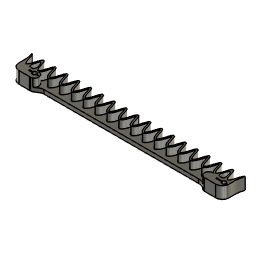
I2process_waku_8mm_change (Autodesk Fusion 360 design; units mm, degrees)
Autodesk Fusion 360 part; units mm, degrees
(part 1 of 7)
sketch "スケッチ1" plane through (0, 0, 0) normal (0, 0, 1) x (1, 0, 0)
  line L0 (269.5, 8.5) -> (265, 8.5)
  line L1 (265, 8.5) -> (262.5, 6)
  line L2 (262.5, 6) -> (257.5, 6)
  line L3 (257.5, 6) -> (255, 8.5)
  line L4 (255, 8.5) -> (250.5, 8.5)
  line L5 (250.5, 7.5) -> (255, 7.5)
  line L6 (255, 7.5) -> (257.5, 5)
  line L7 (257.5, 5) -> (262.5, 5)
  line L8 (262.5, 5) -> (265, 7.5)
  line L9 (265, 7.5) -> (269.5, 7.5)
  line L10 (269.5187, 10.492) -> (262.5532, 10.492)
  line L11 (257.4467, 10.492) -> (250.4813, 10.492)
  line L12 (250.4813, 9.5109) -> (257.4466, 9.5109)
  line L13 (262.5533, 9.5109) -> (269.5187, 9.5109)
  arc A0 (257.4466, 9.5109) -> (262.5533, 9.5109) centre (260, 10.0015) ccw
  arc A1 (262.5532, 10.492) -> (257.4467, 10.492) centre (260, 10.0015) ccw
  spline S0 degree 5 poles (10, 15) (10.1382, 15.0986) (10.4088, 15.309) (10.7966, 15.6643) (11.2779, 16.2176) (11.8206, 17.0415) (12.3075, 17.9961) (12.7453, 19.0761) (13.1463, 20.2726) (13.5274, 21.5702) (13.9072, 22.9453) (14.3043, 24.3634) (14.7345, 25.777) (15.2088, 27.1236) (15.7302, 28.3211) (16.2937, 29.2738) (16.8886, 29.8918) (17.5, 30.1073) (18.1114, 29.8918) (18.7063, 29.2738) (19.2698, 28.3211) (19.7912, 27.1236) (20.2655, 25.777) (20.6957, 24.3634) (21.0928, 22.9453) (21.4726, 21.5702) (21.8537, 20.2726) (22.2547, 19.0761) (22.6925, 17.9961) (23.1794, 17.0415) (23.7221, 16.2176) (24.2034, 15.6643) (24.5912, 15.309) (24.8618, 15.0986) (25, 15) knots 0 0 0 0 0 0 0.033333 0.066667 0.1 0.133333 0.166667 0.2 0.233333 0.266667 0.3 0.333333 0.366667 0.4 0.433333 0.466667 0.5 0.533333 0.566667 0.6 0.633333 0.666667 0.7 0.733333 0.766667 0.8 0.833333 0.866667 0.9 0.933333 0.966667 1 1 1 1 1 1
  spline S1 degree 5 poles (25, 15) (25.1382, 15.0986) (25.4088, 15.309) (25.7966, 15.6643) (26.2779, 16.2176) (26.8206, 17.0415) (27.3075, 17.9961) (27.7453, 19.0761) (28.1463, 20.2726) (28.5274, 21.5702) (28.9072, 22.9453) (29.3043, 24.3634) (29.7345, 25.777) (30.2088, 27.1236) (30.7302, 28.3211) (31.2937, 29.2738) (31.8886, 29.8918) (32.5, 30.1073) (33.1114, 29.8918) (33.7063, 29.2738) (34.2698, 28.3211) (34.7912, 27.1236) (35.2655, 25.777) (35.6957, 24.3634) (36.0928, 22.9453) (36.4726, 21.5702) (36.8537, 20.2726) (37.2547, 19.0761) (37.6925, 17.9961) (38.1794, 17.0415) (38.7221, 16.2176) (39.2034, 15.6643) (39.5912, 15.309) (39.8618, 15.0986) (40, 15) knots 0 0 0 0 0 0 0.033333 0.066667 0.1 0.133333 0.166667 0.2 0.233333 0.266667 0.3 0.333333 0.366667 0.4 0.433333 0.466667 0.5 0.533333 0.566667 0.6 0.633333 0.666667 0.7 0.733333 0.766667 0.8 0.833333 0.866667 0.9 0.933333 0.966667 1 1 1 1 1 1
  spline S2 degree 5 poles (40, 15) (40.1382, 15.0986) (40.4088, 15.309) (40.7966, 15.6643) (41.2779, 16.2176) (41.8206, 17.0415) (42.3075, 17.9961) (42.7453, 19.0761) (43.1463, 20.2726) (43.5274, 21.5702) (43.9072, 22.9453) (44.3043, 24.3634) (44.7345, 25.777) (45.2088, 27.1236) (45.7302, 28.3211) (46.2937, 29.2738) (46.8886, 29.8918) (47.5, 30.1073) (48.1114, 29.8918) (48.7063, 29.2738) (49.2698, 28.3211) (49.7912, 27.1236) (50.2655, 25.777) (50.6957, 24.3634) (51.0928, 22.9453) (51.4726, 21.5702) (51.8537, 20.2726) (52.2547, 19.0761) (52.6925, 17.9961) (53.1794, 17.0415) (53.7221, 16.2176) (54.2034, 15.6643) (54.5912, 15.309) (54.8618, 15.0986) (55, 15) knots 0 0 0 0 0 0 0.033333 0.066667 0.1 0.133333 0.166667 0.2 0.233333 0.266667 0.3 0.333333 0.366667 0.4 0.433333 0.466667 0.5 0.533333 0.566667 0.6 0.633333 0.666667 0.7 0.733333 0.766667 0.8 0.833333 0.866667 0.9 0.933333 0.966667 1 1 1 1 1 1
  spline S3 degree 5 poles (55, 15) (55.1382, 15.0986) (55.4088, 15.309) (55.7966, 15.6643) (56.2779, 16.2176) (56.8206, 17.0415) (57.3075, 17.9961) (57.7453, 19.0761) (58.1463, 20.2726) (58.5274, 21.5702) (58.9072, 22.9453) (59.3043, 24.3634) (59.7345, 25.777) (60.2088, 27.1236) (60.7302, 28.3211) (61.2937, 29.2738) (61.8886, 29.8918) (62.5, 30.1073) (63.1114, 29.8918) (63.7063, 29.2738) (64.2698, 28.3211) (64.7912, 27.1236) (65.2655, 25.777) (65.6957, 24.3634) (66.0928, 22.9453) (66.4726, 21.5702) (66.8537, 20.2726) (67.2547, 19.0761) (67.6925, 17.9961) (68.1794, 17.0415) (68.7221, 16.2176) (69.2034, 15.6643) (69.5912, 15.309) (69.8618, 15.0986) (70, 15) knots 0 0 0 0 0 0 0.033333 0.066667 0.1 0.133333 0.166667 0.2 0.233333 0.266667 0.3 0.333333 0.366667 0.4 0.433333 0.466667 0.5 0.533333 0.566667 0.6 0.633333 0.666667 0.7 0.733333 0.766667 0.8 0.833333 0.866667 0.9 0.933333 0.966667 1 1 1 1 1 1
  spline S4 degree 5 poles (70, 15) (70.1382, 15.0986) (70.4088, 15.309) (70.7966, 15.6643) (71.2779, 16.2176) (71.8206, 17.0415) (72.3075, 17.9961) (72.7453, 19.0761) (73.1463, 20.2726) (73.5274, 21.5702) (73.9072, 22.9453) (74.3043, 24.3634) (74.7345, 25.777) (75.2088, 27.1236) (75.7302, 28.3211) (76.2937, 29.2738) (76.8886, 29.8918) (77.5, 30.1073) (78.1114, 29.8918) (78.7063, 29.2738) (79.2698, 28.3211) (79.7912, 27.1236) (80.2655, 25.777) (80.6957, 24.3634) (81.0928, 22.9453) (81.4726, 21.5702) (81.8537, 20.2726) (82.2547, 19.0761) (82.6925, 17.9961) (83.1794, 17.0415) (83.7221, 16.2176) (84.2034, 15.6643) (84.5912, 15.309) (84.8618, 15.0986) (85, 15) knots 0 0 0 0 0 0 0.033333 0.066667 0.1 0.133333 0.166667 0.2 0.233333 0.266667 0.3 0.333333 0.366667 0.4 0.433333 0.466667 0.5 0.533333 0.566667 0.6 0.633333 0.666667 0.7 0.733333 0.766667 0.8 0.833333 0.866667 0.9 0.933333 0.966667 1 1 1 1 1 1
  spline S5 degree 5 poles (85, 15) (85.1382, 15.0986) (85.4088, 15.309) (85.7966, 15.6643) (86.2779, 16.2176) (86.8206, 17.0415) (87.3075, 17.9961) (87.7453, 19.0761) (88.1463, 20.2726) (88.5274, 21.5702) (88.9072, 22.9453) (89.3043, 24.3634) (89.7345, 25.777) (90.2088, 27.1236) (90.7302, 28.3211) (91.2937, 29.2738) (91.8886, 29.8918) (92.5, 30.1073) (93.1114, 29.8918) (93.7063, 29.2738) (94.2698, 28.3211) (94.7912, 27.1236) (95.2655, 25.777) (95.6957, 24.3634) (96.0928, 22.9453) (96.4726, 21.5702) (96.8537, 20.2726) (97.2547, 19.0761) (97.6925, 17.9961) (98.1794, 17.0415) (98.7221, 16.2176) (99.2034, 15.6643) (99.5912, 15.309) (99.8618, 15.0986) (100, 15) knots 0 0 0 0 0 0 0.033333 0.066667 0.1 0.133333 0.166667 0.2 0.233333 0.266667 0.3 0.333333 0.366667 0.4 0.433333 0.466667 0.5 0.533333 0.566667 0.6 0.633333 0.666667 0.7 0.733333 0.766667 0.8 0.833333 0.866667 0.9 0.933333 0.966667 1 1 1 1 1 1
  spline S6 degree 5 poles (100, 15) (100.1382, 15.0986) (100.4088, 15.309) (100.7966, 15.6643) (101.2779, 16.2176) (101.8206, 17.0415) (102.3075, 17.9961) (102.7453, 19.0761) (103.1463, 20.2726) (103.5274, 21.5702) (103.9072, 22.9453) (104.3043, 24.3634) (104.7345, 25.777) (105.2088, 27.1236) (105.7302, 28.3211) (106.2937, 29.2738) (106.8886, 29.8918) (107.5, 30.1073) (108.1114, 29.8918) (108.7063, 29.2738) (109.2698, 28.3211) (109.7912, 27.1236) (110.2655, 25.777) (110.6957, 24.3634) (111.0928, 22.9453) (111.4726, 21.5702) (111.8537, 20.2726) (112.2547, 19.0761) (112.6925, 17.9961) (113.1794, 17.0415) (113.7221, 16.2176) (114.2034, 15.6643) (114.5912, 15.309) (114.8618, 15.0986) (115, 15) knots 0 0 0 0 0 0 0.033333 0.066667 0.1 0.133333 0.166667 0.2 0.233333 0.266667 0.3 0.333333 0.366667 0.4 0.433333 0.466667 0.5 0.533333 0.566667 0.6 0.633333 0.666667 0.7 0.733333 0.766667 0.8 0.833333 0.866667 0.9 0.933333 0.966667 1 1 1 1 1 1
  spline S7 degree 5 poles (115, 15) (115.1382, 15.0986) (115.4088, 15.309) (115.7966, 15.6643) (116.2779, 16.2176) (116.8206, 17.0415) (117.3075, 17.9961) (117.7453, 19.0761) (118.1463, 20.2726) (118.5274, 21.5702) (118.9072, 22.9453) (119.3043, 24.3634) (119.7345, 25.777) (120.2088, 27.1236) (120.7302, 28.3211) (121.2937, 29.2738) (121.8886, 29.8918) (122.5, 30.1073) (123.1114, 29.8918) (123.7063, 29.2738) (124.2698, 28.3211) (124.7912, 27.1236) (125.2655, 25.777) (125.6957, 24.3634) (126.0928, 22.9453) (126.4726, 21.5702) (126.8537, 20.2726) (127.2547, 19.0761) (127.6925, 17.9961) (128.1794, 17.0415) (128.7221, 16.2176) (129.2034, 15.6643) (129.5912, 15.309) (129.8618, 15.0986) (130, 15) knots 0 0 0 0 0 0 0.033333 0.066667 0.1 0.133333 0.166667 0.2 0.233333 0.266667 0.3 0.333333 0.366667 0.4 0.433333 0.466667 0.5 0.533333 0.566667 0.6 0.633333 0.666667 0.7 0.733333 0.766667 0.8 0.833333 0.866667 0.9 0.933333 0.966667 1 1 1 1 1 1
  spline S8 degree 5 poles (205, 15) (205.1382, 15.0986) (205.4088, 15.309) (205.7966, 15.6643) (206.2779, 16.2176) (206.8206, 17.0415) (207.3075, 17.9961) (207.7453, 19.0761) (208.1463, 20.2726) (208.5274, 21.5702) (208.9072, 22.9453) (209.3043, 24.3634) (209.7345, 25.777) (210.2088, 27.1236) (210.7302, 28.3211) (211.2937, 29.2738) (211.8886, 29.8918) (212.5, 30.1073) (213.1114, 29.8918) (213.7063, 29.2738) (214.2698, 28.3211) (214.7912, 27.1236) (215.2655, 25.777) (215.6957, 24.3634) (216.0928, 22.9453) (216.4726, 21.5702) (216.8537, 20.2726) (217.2547, 19.0761) (217.6925, 17.9961) (218.1794, 17.0415) (218.7221, 16.2176) (219.2034, 15.6643) (219.5912, 15.309) (219.8618, 15.0986) (220, 15) knots 0 0 0 0 0 0 0.033333 0.066667 0.1 0.133333 0.166667 0.2 0.233333 0.266667 0.3 0.333333 0.366667 0.4 0.433333 0.466667 0.5 0.533333 0.566667 0.6 0.633333 0.666667 0.7 0.733333 0.766667 0.8 0.833333 0.866667 0.9 0.933333 0.966667 1 1 1 1 1 1
  spline S9 degree 5 poles (145, 15) (145.1382, 15.0986) (145.4088, 15.309) (145.7966, 15.6643) (146.2779, 16.2176) (146.8206, 17.0415) (147.3075, 17.9961) (147.7453, 19.0761) (148.1463, 20.2726) (148.5274, 21.5702) (148.9072, 22.9453) (149.3043, 24.3634) (149.7345, 25.777) (150.2088, 27.1236) (150.7302, 28.3211) (151.2937, 29.2738) (151.8886, 29.8918) (152.5, 30.1073) (153.1114, 29.8918) (153.7063, 29.2738) (154.2698, 28.3211) (154.7912, 27.1236) (155.2655, 25.777) (155.6957, 24.3634) (156.0928, 22.9453) (156.4726, 21.5702) (156.8537, 20.2726) (157.2547, 19.0761) (157.6925, 17.9961) (158.1794, 17.0415) (158.7221, 16.2176) (159.2034, 15.6643) (159.5912, 15.309) (159.8618, 15.0986) (160, 15) knots 0 0 0 0 0 0 0.033333 0.066667 0.1 0.133333 0.166667 0.2 0.233333 0.266667 0.3 0.333333 0.366667 0.4 0.433333 0.466667 0.5 0.533333 0.566667 0.6 0.633333 0.666667 0.7 0.733333 0.766667 0.8 0.833333 0.866667 0.9 0.933333 0.966667 1 1 1 1 1 1
  spline S10 degree 5 poles (175, 15) (175.1382, 15.0986) (175.4088, 15.309) (175.7966, 15.6643) (176.2779, 16.2176) (176.8206, 17.0415) (177.3075, 17.9961) (177.7453, 19.0761) (178.1463, 20.2726) (178.5274, 21.5702) (178.9072, 22.9453) (179.3043, 24.3634) (179.7345, 25.777) (180.2088, 27.1236) (180.7302, 28.3211) (181.2937, 29.2738) (181.8886, 29.8918) (182.5, 30.1073) (183.1114, 29.8918) (183.7063, 29.2738) (184.2698, 28.3211) (184.7912, 27.1236) (185.2655, 25.777) (185.6957, 24.3634) (186.0928, 22.9453) (186.4726, 21.5702) (186.8537, 20.2726) (187.2547, 19.0761) (187.6925, 17.9961) (188.1794, 17.0415) (188.7221, 16.2176) (189.2034, 15.6643) (189.5912, 15.309) (189.8618, 15.0986) (190, 15) knots 0 0 0 0 0 0 0.033333 0.066667 0.1 0.133333 0.166667 0.2 0.233333 0.266667 0.3 0.333333 0.366667 0.4 0.433333 0.466667 0.5 0.533333 0.566667 0.6 0.633333 0.666667 0.7 0.733333 0.766667 0.8 0.833333 0.866667 0.9 0.933333 0.966667 1 1 1 1 1 1
  spline S11 degree 5 poles (220, 15) (220.1382, 15.0986) (220.4088, 15.309) (220.7966, 15.6643) (221.2779, 16.2176) (221.8206, 17.0415) (222.3075, 17.9961) (222.7453, 19.0761) (223.1463, 20.2726) (223.5274, 21.5702) (223.9072, 22.9453) (224.3043, 24.3634) (224.7345, 25.777) (225.2088, 27.1236) (225.7302, 28.3211) (226.2937, 29.2738) (226.8886, 29.8918) (227.5, 30.1073) (228.1114, 29.8918) (228.7063, 29.2738) (229.2698, 28.3211) (229.7912, 27.1236) (230.2655, 25.777) (230.6957, 24.3634) (231.0928, 22.9453) (231.4726, 21.5702) (231.8537, 20.2726) (232.2547, 19.0761) (232.6925, 17.9961) (233.1794, 17.0415) (233.7221, 16.2176) (234.2034, 15.6643) (234.5912, 15.309) (234.8618, 15.0986) (235, 15) knots 0 0 0 0 0 0 0.033333 0.066667 0.1 0.133333 0.166667 0.2 0.233333 0.266667 0.3 0.333333 0.366667 0.4 0.433333 0.466667 0.5 0.533333 0.566667 0.6 0.633333 0.666667 0.7 0.733333 0.766667 0.8 0.833333 0.866667 0.9 0.933333 0.966667 1 1 1 1 1 1
  spline S12 degree 5 poles (190, 15) (190.1382, 15.0986) (190.4088, 15.309) (190.7966, 15.6643) (191.2779, 16.2176) (191.8206, 17.0415) (192.3075, 17.9961) (192.7453, 19.0761) (193.1463, 20.2726) (193.5274, 21.5702) (193.9072, 22.9453) (194.3043, 24.3634) (194.7345, 25.777) (195.2088, 27.1236) (195.7302, 28.3211) (196.2937, 29.2738) (196.8886, 29.8918) (197.5, 30.1073) (198.1114, 29.8918) (198.7063, 29.2738) (199.2698, 28.3211) (199.7912, 27.1236) (200.2655, 25.777) (200.6957, 24.3634) (201.0928, 22.9453) (201.4726, 21.5702) (201.8537, 20.2726) (202.2547, 19.0761) (202.6925, 17.9961) (203.1794, 17.0415) (203.7221, 16.2176) (204.2034, 15.6643) (204.5912, 15.309) (204.8618, 15.0986) (205, 15) knots 0 0 0 0 0 0 0.033333 0.066667 0.1 0.133333 0.166667 0.2 0.233333 0.266667 0.3 0.333333 0.366667 0.4 0.433333 0.466667 0.5 0.533333 0.566667 0.6 0.633333 0.666667 0.7 0.733333 0.766667 0.8 0.833333 0.866667 0.9 0.933333 0.966667 1 1 1 1 1 1
  spline S13 degree 5 poles (235, 15) (235.1382, 15.0986) (235.4088, 15.309) (235.7966, 15.6643) (236.2779, 16.2176) (236.8206, 17.0415) (237.3075, 17.9961) (237.7453, 19.0761) (238.1463, 20.2726) (238.5274, 21.5702) (238.9072, 22.9453) (239.3043, 24.3634) (239.7345, 25.777) (240.2088, 27.1236) (240.7302, 28.3211) (241.2937, 29.2738) (241.8886, 29.8918) (242.5, 30.1073) (243.1114, 29.8918) (243.7063, 29.2738) (244.2698, 28.3211) (244.7912, 27.1236) (245.2655, 25.777) (245.6957, 24.3634) (246.0928, 22.9453) (246.4726, 21.5702) (246.8537, 20.2726) (247.2547, 19.0761) (247.6925, 17.9961) (248.1794, 17.0415) (248.7221, 16.2176) (249.2034, 15.6643) (249.5912, 15.309) (249.8618, 15.0986) (250, 15) knots 0 0 0 0 0 0 0.033333 0.066667 0.1 0.133333 0.166667 0.2 0.233333 0.266667 0.3 0.333333 0.366667 0.4 0.433333 0.466667 0.5 0.533333 0.566667 0.6 0.633333 0.666667 0.7 0.733333 0.766667 0.8 0.833333 0.866667 0.9 0.933333 0.966667 1 1 1 1 1 1
  spline S14 degree 5 poles (160, 15) (160.1382, 15.0986) (160.4088, 15.309) (160.7966, 15.6643) (161.2779, 16.2176) (161.8206, 17.0415) (162.3075, 17.9961) (162.7453, 19.0761) (163.1463, 20.2726) (163.5274, 21.5702) (163.9072, 22.9453) (164.3043, 24.3634) (164.7345, 25.777) (165.2088, 27.1236) (165.7302, 28.3211) (166.2937, 29.2738) (166.8886, 29.8918) (167.5, 30.1073) (168.1114, 29.8918) (168.7063, 29.2738) (169.2698, 28.3211) (169.7912, 27.1236) (170.2655, 25.777) (170.6957, 24.3634) (171.0928, 22.9453) (171.4726, 21.5702) (171.8537, 20.2726) (172.2547, 19.0761) (172.6925, 17.9961) (173.1794, 17.0415) (173.7221, 16.2176) (174.2034, 15.6643) (174.5912, 15.309) (174.8618, 15.0986) (175, 15) knots 0 0 0 0 0 0 0.033333 0.066667 0.1 0.133333 0.166667 0.2 0.233333 0.266667 0.3 0.333333 0.366667 0.4 0.433333 0.466667 0.5 0.533333 0.566667 0.6 0.633333 0.666667 0.7 0.733333 0.766667 0.8 0.833333 0.866667 0.9 0.933333 0.966667 1 1 1 1 1 1
  spline S15 degree 5 poles (130, 15) (130.1382, 15.0986) (130.4088, 15.309) (130.7966, 15.6643) (131.2779, 16.2176) (131.8206, 17.0415) (132.3075, 17.9961) (132.7453, 19.0761) (133.1463, 20.2726) (133.5274, 21.5702) (133.9072, 22.9453) (134.3043, 24.3634) (134.7345, 25.777) (135.2088, 27.1236) (135.7302, 28.3211) (136.2937, 29.2738) (136.8886, 29.8918) (137.5, 30.1073) (138.1114, 29.8918) (138.7063, 29.2738) (139.2698, 28.3211) (139.7912, 27.1236) (140.2655, 25.777) (140.6957, 24.3634) (141.0928, 22.9453) (141.4726, 21.5702) (141.8537, 20.2726) (142.2547, 19.0761) (142.6925, 17.9961) (143.1794, 17.0415) (143.7221, 16.2176) (144.2034, 15.6643) (144.5912, 15.309) (144.8618, 15.0986) (145, 15) knots 0 0 0 0 0 0 0.033333 0.066667 0.1 0.133333 0.166667 0.2 0.233333 0.266667 0.3 0.333333 0.366667 0.4 0.433333 0.466667 0.5 0.533333 0.566667 0.6 0.633333 0.666667 0.7 0.733333 0.766667 0.8 0.833333 0.866667 0.9 0.933333 0.966667 1 1 1 1 1 1
  spline S16 degree 5 poles (250, 15) (250.1382, 15.0986) (250.4088, 15.309) (250.7966, 15.6643) (251.2779, 16.2176) (251.8206, 17.0415) (252.3075, 17.9961) (252.7453, 19.0761) (253.1463, 20.2726) (253.5274, 21.5702) (253.9072, 22.9453) (254.3043, 24.3634) (254.7345, 25.777) (255.2088, 27.1236) (255.7302, 28.3211) (256.2937, 29.2738) (256.8886, 29.8918) (257.5, 30.1073) (258.1114, 29.8918) (258.7063, 29.2738) (259.2698, 28.3211) (259.7912, 27.1236) (260.2655, 25.777) (260.6957, 24.3634) (261.0928, 22.9453) (261.4726, 21.5702) (261.8537, 20.2726) (262.2547, 19.0761) (262.6925, 17.9961) (263.1794, 17.0415) (263.7221, 16.2176) (264.2034, 15.6643) (264.5912, 15.309) (264.8618, 15.0986) (265, 15) knots 0 0 0 0 0 0 0.033333 0.066667 0.1 0.133333 0.166667 0.2 0.233333 0.266667 0.3 0.333333 0.366667 0.4 0.433333 0.466667 0.5 0.533333 0.566667 0.6 0.633333 0.666667 0.7 0.733333 0.766667 0.8 0.833333 0.866667 0.9 0.933333 0.966667 1 1 1 1 1 1
  arc A2 (269.5, 7.5) -> (269.5, 8.5) centre (269.5, 8) ccw
  arc A3 (269.5, 9.5109) -> (269.5, 10.492) centre (269.5093, 10.0015) ccw
  arc A4 (250.5, 8.5) -> (250.5, 7.5) centre (250.5, 8) ccw
  arc A5 (250.5, 10.492) -> (250.5, 9.5109) centre (250.4907, 10.0015) ccw
  arc A6 (267, 3) -> (267, 15) centre (267, 9) ccw
  line L14 (267, 15) -> (265, 15)
  line L15 (10, 7.5) -> (12.5, 5)
  arc A7 (5.5, 10.492) -> (5.5, 9.5109) centre (5.4907, 10.0015) ccw
  arc A8 (17.5532, 10.492) -> (12.4467, 10.492) centre (15, 10.0015) ccw
  arc A9 (24.5, 7.5) -> (24.5, 8.5) centre (24.5, 8) ccw
  line L16 (17.5, 5) -> (20, 7.5)
  arc A10 (24.5, 9.5109) -> (24.5, 10.492) centre (24.5093, 10.0015) ccw
  arc A11 (5.5, 8.5) -> (5.5, 7.5) centre (5.5, 8) ccw
  line L17 (5.5, 7.5) -> (10, 7.5)
  line L18 (12.4467, 10.492) -> (5.4813, 10.492)
  line L19 (12.5, 6) -> (10, 8.5)
  arc A12 (12.4466, 9.5109) -> (17.5533, 9.5109) centre (15, 10.0015) ccw
  line L20 (17.5533, 9.5109) -> (24.5187, 9.5109)
  line L21 (17.5, 6) -> (12.5, 6)
  line L22 (12.5, 5) -> (17.5, 5)
  line L23 (20, 7.5) -> (24.5, 7.5)
  line L24 (24.5, 8.5) -> (20, 8.5)
  line L25 (5.4813, 9.5109) -> (12.4466, 9.5109)
  line L26 (10, 8.5) -> (5.5, 8.5)
  line L27 (24.5187, 10.492) -> (17.5532, 10.492)
  line L28 (20, 8.5) -> (17.5, 6)
  line L29 (10, 15) -> (8, 15)
  arc A13 (8, 15) -> (8, 3) centre (8, 9) ccw
  line L30 (8, 3) -> (267, 3)
  point P0 (260, 10.0015)
  point P1 (12.5, 18.5)
  point P2 (15, 26.5)
  point P3 (17.5, 30)
  point P4 (20, 26.5)
  point P5 (22.5, 18.5)
  point P6 (30, 26.5)
  point P7 (27.5, 18.5)
  point P8 (32.5, 30)
  point P9 (37.5, 18.5)
  point P10 (35, 26.5)
  point P11 (60, 26.5)
  point P12 (57.5, 18.5)
  point P13 (65, 26.5)
  point P14 (67.5, 18.5)
  point P15 (62.5, 30)
  point P16 (45, 26.5)
  point P17 (42.5, 18.5)
  point P18 (47.5, 30)
  point P19 (52.5, 18.5)
  point P20 (50, 26.5)
  point P21 (127.5, 18.5)
  point P22 (105, 26.5)
  point P23 (125, 26.5)
  point P24 (122.5, 30)
  point P25 (112.5, 18.5)
  point P26 (120, 26.5)
  point P27 (110, 26.5)
  point P28 (117.5, 18.5)
  point P29 (107.5, 30)
  point P30 (102.5, 18.5)
  point P31 (90, 26.5)
  point P32 (87.5, 18.5)
  point P33 (95, 26.5)
  point P34 (97.5, 18.5)
  point P35 (92.5, 30)
  point P36 (75, 26.5)
  point P37 (72.5, 18.5)
  point P38 (77.5, 30)
  point P39 (82.5, 18.5)
  point P40 (80, 26.5)
  point P41 (187.5, 18.5)
  point P42 (165, 26.5)
  point P43 (185, 26.5)
  point P44 (182.5, 30)
  point P45 (172.5, 18.5)
  point P46 (180, 26.5)
  point P47 (170, 26.5)
  point P48 (177.5, 18.5)
  point P49 (167.5, 30)
  point P50 (162.5, 18.5)
  point P51 (212.5, 30)
  point P52 (192.5, 18.5)
  point P53 (195, 26.5)
  point P54 (200, 26.5)
  point P55 (197.5, 30)
  point P56 (202.5, 18.5)
  point P57 (150, 26.5)
  point P58 (147.5, 18.5)
  point P59 (155, 26.5)
  point P60 (157.5, 18.5)
  point P61 (152.5, 30)
  point P62 (217.5, 18.5)
  point P63 (210, 26.5)
  point P64 (207.5, 18.5)
  point P65 (215, 26.5)
  point P66 (237.5, 18.5)
  point P67 (227.5, 30)
  point P68 (222.5, 18.5)
  point P69 (230, 26.5)
  point P70 (135, 26.5)
  point P71 (132.5, 18.5)
  point P72 (137.5, 30)
  point P73 (142.5, 18.5)
  point P74 (140, 26.5)
  point P75 (247.5, 18.5)
  point P76 (232.5, 18.5)
  point P77 (240, 26.5)
  point P78 (225, 26.5)
  point P79 (245, 26.5)
  point P80 (242.5, 30)
  point P81 (255, 26.5)
  point P82 (262.5, 18.5)
  point P83 (260, 26.5)
  point P84 (252.5, 18.5)
  point P85 (257.5, 30)
  point P86 (15, 10.0015)
  point P87 (22, 9)
  dimension "d4" = 5.2
  dimension "d15" = 2.6
  dimension "d17" = 5.2
  dimension "d18" = 2.6
  constraint coincident P0 A0.centre
  constraint horizontal L10
  constraint horizontal L12
  constraint parallel L0 L12
  constraint parallel L0 L2
  constraint parallel L2 L4
  constraint parallel L3 L6
  constraint parallel L5 L7
  constraint perpendicular L3 L8
  constraint parallel L5 L9
  constraint coincident L10.end A0
  constraint collinear L10 L11
  constraint collinear L12 L13
  constraint concentric A0 A1
  constraint coincident L10 A3.end
  constraint coincident L13 A3.start
  constraint coincident L11 A5.start
  constraint coincident L12 A5.end
  constraint coincident A5 L12.start
  constraint coincident A5 L11.end
  constraint coincident A3 L13.end
  constraint coincident A3 L10.start
  constraint tangent A6 L14
  constraint coincident P86 A8.centre
  constraint horizontal L27
  constraint horizontal L25
  constraint parallel L24 L25
  constraint parallel L21 L24
  constraint parallel L21 L26
  constraint parallel L15 L19
  constraint parallel L17 L22
  constraint perpendicular L16 L19
  constraint parallel L17 L23
  constraint coincident A8.start A12
  constraint collinear L18 L27
  constraint collinear L20 L25
  constraint concentric A8 A12
  constraint coincident A10.end L27
  constraint coincident A10.start L20
  constraint coincident A7.start L18
  constraint coincident A7.end L25
  constraint coincident L25.start A7
  constraint coincident L18.end A7
  constraint coincident L20.end A10
  constraint coincident L27.start A10
  constraint horizontal L29
  constraint tangent L29 A13
  constraint tangent A6 L30
  measures "d4" diameter of A0
  measures "d15" radius of A0
  measures "d17" diameter of A12
  measures "d18" radius of A12
sketch "スケッチ4" plane through (0, 0, 0) normal (0, 0, 1) x (1, 0, 0)
sketch "スケッチ5" plane through (0, 0, 20) normal (0, 0, 1) x (-1, 0, 0)
  arc A0 (-250.5, -8.5) -> (-250.5, -7.5) centre (-250.5, -8) ccw
  line L0 (-250.5, -8.5) -> (-255, -8.5)
  line L1 (-255, -8.5) -> (-257.5, -6)
  line L2 (-257.5, -6) -> (-262.5, -6)
  line L3 (-262.5, -6) -> (-265, -8.5)
  line L4 (-265, -8.5) -> (-269.5, -8.5)
  arc A1 (-269.5, -7.5) -> (-269.5, -8.5) centre (-269.5, -8) ccw
  line L5 (-269.5, -7.5) -> (-265, -7.5)
  line L6 (-265, -7.5) -> (-262.5, -5)
  line L7 (-262.5, -5) -> (-257.5, -5)
  line L8 (-257.5, -5) -> (-255, -7.5)
  line L9 (-255, -7.5) -> (-250.5, -7.5)
  arc A2 (-250.5, -10.492) -> (-250.5, -9.5109) centre (-250.4907, -10.0015) ccw
  line L10 (-250.5, -10.492) -> (-257.4467, -10.492)
  arc A3 (-262.5532, -10.492) -> (-257.4467, -10.492) centre (-260, -10.0015) ccw
  line L11 (-262.5532, -10.492) -> (-269.5, -10.492)
  arc A4 (-269.5, -9.5109) -> (-269.5, -10.492) centre (-269.5093, -10.0015) ccw
  line L12 (-269.5, -9.5109) -> (-262.5533, -9.5109)
  arc A5 (-257.4466, -9.5109) -> (-262.5533, -9.5109) centre (-260, -10.0015) ccw
  line L13 (-257.4466, -9.5109) -> (-250.5, -9.5109)
  line L14 (-17.5, -6) -> (-20, -8.5)
  line L15 (-20, -8.5) -> (-24.5, -8.5)
  arc A6 (-24.5, -7.5) -> (-24.5, -8.5) centre (-24.5, -8) ccw
  line L16 (-24.5, -7.5) -> (-20, -7.5)
  line L17 (-20, -7.5) -> (-17.5, -5)
  line L18 (-17.5, -5) -> (-12.5, -5)
  line L19 (-12.5, -5) -> (-10, -7.5)
  line L20 (-10, -7.5) -> (-5.5, -7.5)
  arc A7 (-5.5, -8.5) -> (-5.5, -7.5) centre (-5.5, -8) ccw
  line L21 (-5.5, -8.5) -> (-10, -8.5)
  line L22 (-10, -8.5) -> (-12.5, -6)
  line L23 (-12.5, -6) -> (-17.5, -6)
  arc A8 (-24.5, -9.5109) -> (-24.5, -10.492) centre (-24.5093, -10.0015) ccw
  line L24 (-24.5, -9.5109) -> (-17.5533, -9.5109)
  arc A9 (-12.4466, -9.5109) -> (-17.5533, -9.5109) centre (-15, -10.0015) ccw
  line L25 (-12.4466, -9.5109) -> (-5.5, -9.5109)
  arc A10 (-5.5, -10.492) -> (-5.5, -9.5109) centre (-5.4907, -10.0015) ccw
  line L26 (-5.5, -10.492) -> (-12.4467, -10.492)
  arc A11 (-17.5532, -10.492) -> (-12.4467, -10.492) centre (-15, -10.0015) ccw
  line L27 (-17.5532, -10.492) -> (-24.5, -10.492)
  line L28 (-10, -15) -> (-8, -15)
  arc A12 (-8, -15) -> (-8, -3) centre (-8, -9) ccw
  line L29 (-8, -3) -> (-267, -3)
  arc A13 (-267, -3) -> (-267, -15) centre (-267, -9) ccw
  line L30 (-267, -15) -> (-265, -15)
  spline S0 degree 5 poles (-265, -15) (-264.8618, -15.0986) (-264.5912, -15.309) (-264.2034, -15.6643) (-263.7221, -16.2176) (-263.1794, -17.0415) (-262.6925, -17.9961) (-262.2547, -19.0761) (-261.8537, -20.2726) (-261.4726, -21.5702) (-261.0928, -22.9453) (-260.6957, -24.3634) (-260.2655, -25.777) (-259.7912, -27.1236) (-259.2698, -28.3211) (-258.7063, -29.2738) (-258.1114, -29.8918) (-257.5, -30.1073) (-256.8886, -29.8918) (-256.2937, -29.2738) (-255.7302, -28.3211) (-255.2088, -27.1236) (-254.7345, -25.777) (-254.3043, -24.3634) (-253.9072, -22.9453) (-253.5274, -21.5702) (-253.1463, -20.2726) (-252.7453, -19.0761) (-252.3075, -17.9961) (-251.8206, -17.0415) (-251.2779, -16.2176) (-250.7966, -15.6643) (-250.4088, -15.309) (-250.1382, -15.0986) (-250, -15) knots -1 -1 -1 -1 -1 -1 -0.966667 -0.933333 -0.9 -0.866667 -0.833333 -0.8 -0.766667 -0.733333 -0.7 -0.666667 -0.633333 -0.6 -0.566667 -0.533333 -0.5 -0.466667 -0.433333 -0.4 -0.366667 -0.333333 -0.3 -0.266667 -0.233333 -0.2 -0.166667 -0.133333 -0.1 -0.066667 -0.033333 0 0 0 0 0 0
  spline S1 degree 5 poles (-250, -15) (-249.8618, -15.0986) (-249.5912, -15.309) (-249.2034, -15.6643) (-248.7221, -16.2176) (-248.1794, -17.0415) (-247.6925, -17.9961) (-247.2547, -19.0761) (-246.8537, -20.2726) (-246.4726, -21.5702) (-246.0928, -22.9453) (-245.6957, -24.3634) (-245.2655, -25.777) (-244.7912, -27.1236) (-244.2698, -28.3211) (-243.7063, -29.2738) (-243.1114, -29.8918) (-242.5, -30.1073) (-241.8886, -29.8918) (-241.2937, -29.2738) (-240.7302, -28.3211) (-240.2088, -27.1236) (-239.7345, -25.777) (-239.3043, -24.3634) (-238.9072, -22.9453) (-238.5274, -21.5702) (-238.1463, -20.2726) (-237.7453, -19.0761) (-237.3075, -17.9961) (-236.8206, -17.0415) (-236.2779, -16.2176) (-235.7966, -15.6643) (-235.4088, -15.309) (-235.1382, -15.0986) (-235, -15) knots -1 -1 -1 -1 -1 -1 -0.966667 -0.933333 -0.9 -0.866667 -0.833333 -0.8 -0.766667 -0.733333 -0.7 -0.666667 -0.633333 -0.6 -0.566667 -0.533333 -0.5 -0.466667 -0.433333 -0.4 -0.366667 -0.333333 -0.3 -0.266667 -0.233333 -0.2 -0.166667 -0.133333 -0.1 -0.066667 -0.033333 0 0 0 0 0 0
  spline S2 degree 5 poles (-235, -15) (-234.8618, -15.0986) (-234.5912, -15.309) (-234.2034, -15.6643) (-233.7221, -16.2176) (-233.1794, -17.0415) (-232.6925, -17.9961) (-232.2547, -19.0761) (-231.8537, -20.2726) (-231.4726, -21.5702) (-231.0928, -22.9453) (-230.6957, -24.3634) (-230.2655, -25.777) (-229.7912, -27.1236) (-229.2698, -28.3211) (-228.7063, -29.2738) (-228.1114, -29.8918) (-227.5, -30.1073) (-226.8886, -29.8918) (-226.2937, -29.2738) (-225.7302, -28.3211) (-225.2088, -27.1236) (-224.7345, -25.777) (-224.3043, -24.3634) (-223.9072, -22.9453) (-223.5274, -21.5702) (-223.1463, -20.2726) (-222.7453, -19.0761) (-222.3075, -17.9961) (-221.8206, -17.0415) (-221.2779, -16.2176) (-220.7966, -15.6643) (-220.4088, -15.309) (-220.1382, -15.0986) (-220, -15) knots -1 -1 -1 -1 -1 -1 -0.966667 -0.933333 -0.9 -0.866667 -0.833333 -0.8 -0.766667 -0.733333 -0.7 -0.666667 -0.633333 -0.6 -0.566667 -0.533333 -0.5 -0.466667 -0.433333 -0.4 -0.366667 -0.333333 -0.3 -0.266667 -0.233333 -0.2 -0.166667 -0.133333 -0.1 -0.066667 -0.033333 0 0 0 0 0 0
  spline S3 degree 5 poles (-220, -15) (-219.8618, -15.0986) (-219.5912, -15.309) (-219.2034, -15.6643) (-218.7221, -16.2176) (-218.1794, -17.0415) (-217.6925, -17.9961) (-217.2547, -19.0761) (-216.8537, -20.2726) (-216.4726, -21.5702) (-216.0928, -22.9453) (-215.6957, -24.3634) (-215.2655, -25.777) (-214.7912, -27.1236) (-214.2698, -28.3211) (-213.7063, -29.2738) (-213.1114, -29.8918) (-212.5, -30.1073) (-211.8886, -29.8918) (-211.2937, -29.2738) (-210.7302, -28.3211) (-210.2088, -27.1236) (-209.7345, -25.777) (-209.3043, -24.3634) (-208.9072, -22.9453) (-208.5274, -21.5702) (-208.1463, -20.2726) (-207.7453, -19.0761) (-207.3075, -17.9961) (-206.8206, -17.0415) (-206.2779, -16.2176) (-205.7966, -15.6643) (-205.4088, -15.309) (-205.1382, -15.0986) (-205, -15) knots -1 -1 -1 -1 -1 -1 -0.966667 -0.933333 -0.9 -0.866667 -0.833333 -0.8 -0.766667 -0.733333 -0.7 -0.666667 -0.633333 -0.6 -0.566667 -0.533333 -0.5 -0.466667 -0.433333 -0.4 -0.366667 -0.333333 -0.3 -0.266667 -0.233333 -0.2 -0.166667 -0.133333 -0.1 -0.066667 -0.033333 0 0 0 0 0 0
  spline S4 degree 5 poles (-205, -15) (-204.8618, -15.0986) (-204.5912, -15.309) (-204.2034, -15.6643) (-203.7221, -16.2176) (-203.1794, -17.0415) (-202.6925, -17.9961) (-202.2547, -19.0761) (-201.8537, -20.2726) (-201.4726, -21.5702) (-201.0928, -22.9453) (-200.6957, -24.3634) (-200.2655, -25.777) (-199.7912, -27.1236) (-199.2698, -28.3211) (-198.7063, -29.2738) (-198.1114, -29.8918) (-197.5, -30.1073) (-196.8886, -29.8918) (-196.2937, -29.2738) (-195.7302, -28.3211) (-195.2088, -27.1236) (-194.7345, -25.777) (-194.3043, -24.3634) (-193.9072, -22.9453) (-193.5274, -21.5702) (-193.1463, -20.2726) (-192.7453, -19.0761) (-192.3075, -17.9961) (-191.8206, -17.0415) (-191.2779, -16.2176) (-190.7966, -15.6643) (-190.4088, -15.309) (-190.1382, -15.0986) (-190, -15) knots -1 -1 -1 -1 -1 -1 -0.966667 -0.933333 -0.9 -0.866667 -0.833333 -0.8 -0.766667 -0.733333 -0.7 -0.666667 -0.633333 -0.6 -0.566667 -0.533333 -0.5 -0.466667 -0.433333 -0.4 -0.366667 -0.333333 -0.3 -0.266667 -0.233333 -0.2 -0.166667 -0.133333 -0.1 -0.066667 -0.033333 0 0 0 0 0 0
  spline S5 degree 5 poles (-190, -15) (-189.8618, -15.0986) (-189.5912, -15.309) (-189.2034, -15.6643) (-188.7221, -16.2176) (-188.1794, -17.0415) (-187.6925, -17.9961) (-187.2547, -19.0761) (-186.8537, -20.2726) (-186.4726, -21.5702) (-186.0928, -22.9453) (-185.6957, -24.3634) (-185.2655, -25.777) (-184.7912, -27.1236) (-184.2698, -28.3211) (-183.7063, -29.2738) (-183.1114, -29.8918) (-182.5, -30.1073) (-181.8886, -29.8918) (-181.2937, -29.2738) (-180.7302, -28.3211) (-180.2088, -27.1236) (-179.7345, -25.777) (-179.3043, -24.3634) (-178.9072, -22.9453) (-178.5274, -21.5702) (-178.1463, -20.2726) (-177.7453, -19.0761) (-177.3075, -17.9961) (-176.8206, -17.0415) (-176.2779, -16.2176) (-175.7966, -15.6643) (-175.4088, -15.309) (-175.1382, -15.0986) (-175, -15) knots -1 -1 -1 -1 -1 -1 -0.966667 -0.933333 -0.9 -0.866667 -0.833333 -0.8 -0.766667 -0.733333 -0.7 -0.666667 -0.633333 -0.6 -0.566667 -0.533333 -0.5 -0.466667 -0.433333 -0.4 -0.366667 -0.333333 -0.3 -0.266667 -0.233333 -0.2 -0.166667 -0.133333 -0.1 -0.066667 -0.033333 0 0 0 0 0 0
  spline S6 degree 5 poles (-175, -15) (-174.8618, -15.0986) (-174.5912, -15.309) (-174.2034, -15.6643) (-173.7221, -16.2176) (-173.1794, -17.0415) (-172.6925, -17.9961) (-172.2547, -19.0761) (-171.8537, -20.2726) (-171.4726, -21.5702) (-171.0928, -22.9453) (-170.6957, -24.3634) (-170.2655, -25.777) (-169.7912, -27.1236) (-169.2698, -28.3211) (-168.7063, -29.2738) (-168.1114, -29.8918) (-167.5, -30.1073) (-166.8886, -29.8918) (-166.2937, -29.2738) (-165.7302, -28.3211) (-165.2088, -27.1236) (-164.7345, -25.777) (-164.3043, -24.3634) (-163.9072, -22.9453) (-163.5274, -21.5702) (-163.1463, -20.2726) (-162.7453, -19.0761) (-162.3075, -17.9961) (-161.8206, -17.0415) (-161.2779, -16.2176) (-160.7966, -15.6643) (-160.4088, -15.309) (-160.1382, -15.0986) (-160, -15) knots -1 -1 -1 -1 -1 -1 -0.966667 -0.933333 -0.9 -0.866667 -0.833333 -0.8 -0.766667 -0.733333 -0.7 -0.666667 -0.633333 -0.6 -0.566667 -0.533333 -0.5 -0.466667 -0.433333 -0.4 -0.366667 -0.333333 -0.3 -0.266667 -0.233333 -0.2 -0.166667 -0.133333 -0.1 -0.066667 -0.033333 0 0 0 0 0 0
  spline S7 degree 5 poles (-160, -15) (-159.8618, -15.0986) (-159.5912, -15.309) (-159.2034, -15.6643) (-158.7221, -16.2176) (-158.1794, -17.0415) (-157.6925, -17.9961) (-157.2547, -19.0761) (-156.8537, -20.2726) (-156.4726, -21.5702) (-156.0928, -22.9453) (-155.6957, -24.3634) (-155.2655, -25.777) (-154.7912, -27.1236) (-154.2698, -28.3211) (-153.7063, -29.2738) (-153.1114, -29.8918) (-152.5, -30.1073) (-151.8886, -29.8918) (-151.2937, -29.2738) (-150.7302, -28.3211) (-150.2088, -27.1236) (-149.7345, -25.777) (-149.3043, -24.3634) (-148.9072, -22.9453) (-148.5274, -21.5702) (-148.1463, -20.2726) (-147.7453, -19.0761) (-147.3075, -17.9961) (-146.8206, -17.0415) (-146.2779, -16.2176) (-145.7966, -15.6643) (-145.4088, -15.309) (-145.1382, -15.0986) (-145, -15) knots -1 -1 -1 -1 -1 -1 -0.966667 -0.933333 -0.9 -0.866667 -0.833333 -0.8 -0.766667 -0.733333 -0.7 -0.666667 -0.633333 -0.6 -0.566667 -0.533333 -0.5 -0.466667 -0.433333 -0.4 -0.366667 -0.333333 -0.3 -0.266667 -0.233333 -0.2 -0.166667 -0.133333 -0.1 -0.066667 -0.033333 0 0 0 0 0 0
  spline S8 degree 5 poles (-145, -15) (-144.8618, -15.0986) (-144.5912, -15.309) (-144.2034, -15.6643) (-143.7221, -16.2176) (-143.1794, -17.0415) (-142.6925, -17.9961) (-142.2547, -19.0761) (-141.8537, -20.2726) (-141.4726, -21.5702) (-141.0928, -22.9453) (-140.6957, -24.3634) (-140.2655, -25.777) (-139.7912, -27.1236) (-139.2698, -28.3211) (-138.7063, -29.2738) (-138.1114, -29.8918) (-137.5, -30.1073) (-136.8886, -29.8918) (-136.2937, -29.2738) (-135.7302, -28.3211) (-135.2088, -27.1236) (-134.7345, -25.777) (-134.3043, -24.3634) (-133.9072, -22.9453) (-133.5274, -21.5702) (-133.1463, -20.2726) (-132.7453, -19.0761) (-132.3075, -17.9961) (-131.8206, -17.0415) (-131.2779, -16.2176) (-130.7966, -15.6643) (-130.4088, -15.309) (-130.1382, -15.0986) (-130, -15) knots -1 -1 -1 -1 -1 -1 -0.966667 -0.933333 -0.9 -0.866667 -0.833333 -0.8 -0.766667 -0.733333 -0.7 -0.666667 -0.633333 -0.6 -0.566667 -0.533333 -0.5 -0.466667 -0.433333 -0.4 -0.366667 -0.333333 -0.3 -0.266667 -0.233333 -0.2 -0.166667 -0.133333 -0.1 -0.066667 -0.033333 0 0 0 0 0 0
  spline S9 degree 5 poles (-130, -15) (-129.8618, -15.0986) (-129.5912, -15.309) (-129.2034, -15.6643) (-128.7221, -16.2176) (-128.1794, -17.0415) (-127.6925, -17.9961) (-127.2547, -19.0761) (-126.8537, -20.2726) (-126.4726, -21.5702) (-126.0928, -22.9453) (-125.6957, -24.3634) (-125.2655, -25.777) (-124.7912, -27.1236) (-124.2698, -28.3211) (-123.7063, -29.2738) (-123.1114, -29.8918) (-122.5, -30.1073) (-121.8886, -29.8918) (-121.2937, -29.2738) (-120.7302, -28.3211) (-120.2088, -27.1236) (-119.7345, -25.777) (-119.3043, -24.3634) (-118.9072, -22.9453) (-118.5274, -21.5702) (-118.1463, -20.2726) (-117.7453, -19.0761) (-117.3075, -17.9961) (-116.8206, -17.0415) (-116.2779, -16.2176) (-115.7966, -15.6643) (-115.4088, -15.309) (-115.1382, -15.0986) (-115, -15) knots -1 -1 -1 -1 -1 -1 -0.966667 -0.933333 -0.9 -0.866667 -0.833333 -0.8 -0.766667 -0.733333 -0.7 -0.666667 -0.633333 -0.6 -0.566667 -0.533333 -0.5 -0.466667 -0.433333 -0.4 -0.366667 -0.333333 -0.3 -0.266667 -0.233333 -0.2 -0.166667 -0.133333 -0.1 -0.066667 -0.033333 0 0 0 0 0 0
  spline S10 degree 5 poles (-115, -15) (-114.8618, -15.0986) (-114.5912, -15.309) (-114.2034, -15.6643) (-113.7221, -16.2176) (-113.1794, -17.0415) (-112.6925, -17.9961) (-112.2547, -19.0761) (-111.8537, -20.2726) (-111.4726, -21.5702) (-111.0928, -22.9453) (-110.6957, -24.3634) (-110.2655, -25.777) (-109.7912, -27.1236) (-109.2698, -28.3211) (-108.7063, -29.2738) (-108.1114, -29.8918) (-107.5, -30.1073) (-106.8886, -29.8918) (-106.2937, -29.2738) (-105.7302, -28.3211) (-105.2088, -27.1236) (-104.7345, -25.777) (-104.3043, -24.3634) (-103.9072, -22.9453) (-103.5274, -21.5702) (-103.1463, -20.2726) (-102.7453, -19.0761) (-102.3075, -17.9961) (-101.8206, -17.0415) (-101.2779, -16.2176) (-100.7966, -15.6643) (-100.4088, -15.309) (-100.1382, -15.0986) (-100, -15) knots -1 -1 -1 -1 -1 -1 -0.966667 -0.933333 -0.9 -0.866667 -0.833333 -0.8 -0.766667 -0.733333 -0.7 -0.666667 -0.633333 -0.6 -0.566667 -0.533333 -0.5 -0.466667 -0.433333 -0.4 -0.366667 -0.333333 -0.3 -0.266667 -0.233333 -0.2 -0.166667 -0.133333 -0.1 -0.066667 -0.033333 0 0 0 0 0 0
  spline S11 degree 5 poles (-100, -15) (-99.8618, -15.0986) (-99.5912, -15.309) (-99.2034, -15.6643) (-98.7221, -16.2176) (-98.1794, -17.0415) (-97.6925, -17.9961) (-97.2547, -19.0761) (-96.8537, -20.2726) (-96.4726, -21.5702) (-96.0928, -22.9453) (-95.6957, -24.3634) (-95.2655, -25.777) (-94.7912, -27.1236) (-94.2698, -28.3211) (-93.7063, -29.2738) (-93.1114, -29.8918) (-92.5, -30.1073) (-91.8886, -29.8918) (-91.2937, -29.2738) (-90.7302, -28.3211) (-90.2088, -27.1236) (-89.7345, -25.777) (-89.3043, -24.3634) (-88.9072, -22.9453) (-88.5274, -21.5702) (-88.1463, -20.2726) (-87.7453, -19.0761) (-87.3075, -17.9961) (-86.8206, -17.0415) (-86.2779, -16.2176) (-85.7966, -15.6643) (-85.4088, -15.309) (-85.1382, -15.0986) (-85, -15) knots -1 -1 -1 -1 -1 -1 -0.966667 -0.933333 -0.9 -0.866667 -0.833333 -0.8 -0.766667 -0.733333 -0.7 -0.666667 -0.633333 -0.6 -0.566667 -0.533333 -0.5 -0.466667 -0.433333 -0.4 -0.366667 -0.333333 -0.3 -0.266667 -0.233333 -0.2 -0.166667 -0.133333 -0.1 -0.066667 -0.033333 0 0 0 0 0 0
  spline S12 degree 5 poles (-85, -15) (-84.8618, -15.0986) (-84.5912, -15.309) (-84.2034, -15.6643) (-83.7221, -16.2176) (-83.1794, -17.0415) (-82.6925, -17.9961) (-82.2547, -19.0761) (-81.8537, -20.2726) (-81.4726, -21.5702) (-81.0928, -22.9453) (-80.6957, -24.3634) (-80.2655, -25.777) (-79.7912, -27.1236) (-79.2698, -28.3211) (-78.7063, -29.2738) (-78.1114, -29.8918) (-77.5, -30.1073) (-76.8886, -29.8918) (-76.2937, -29.2738) (-75.7302, -28.3211) (-75.2088, -27.1236) (-74.7345, -25.777) (-74.3043, -24.3634) (-73.9072, -22.9453) (-73.5274, -21.5702) (-73.1463, -20.2726) (-72.7453, -19.0761) (-72.3075, -17.9961) (-71.8206, -17.0415) (-71.2779, -16.2176) (-70.7966, -15.6643) (-70.4088, -15.309) (-70.1382, -15.0986) (-70, -15) knots -1 -1 -1 -1 -1 -1 -0.966667 -0.933333 -0.9 -0.866667 -0.833333 -0.8 -0.766667 -0.733333 -0.7 -0.666667 -0.633333 -0.6 -0.566667 -0.533333 -0.5 -0.466667 -0.433333 -0.4 -0.366667 -0.333333 -0.3 -0.266667 -0.233333 -0.2 -0.166667 -0.133333 -0.1 -0.066667 -0.033333 0 0 0 0 0 0
  spline S13 degree 5 poles (-70, -15) (-69.8618, -15.0986) (-69.5912, -15.309) (-69.2034, -15.6643) (-68.7221, -16.2176) (-68.1794, -17.0415) (-67.6925, -17.9961) (-67.2547, -19.0761) (-66.8537, -20.2726) (-66.4726, -21.5702) (-66.0928, -22.9453) (-65.6957, -24.3634) (-65.2655, -25.777) (-64.7912, -27.1236) (-64.2698, -28.3211) (-63.7063, -29.2738) (-63.1114, -29.8918) (-62.5, -30.1073) (-61.8886, -29.8918) (-61.2937, -29.2738) (-60.7302, -28.3211) (-60.2088, -27.1236) (-59.7345, -25.777) (-59.3043, -24.3634) (-58.9072, -22.9453) (-58.5274, -21.5702) (-58.1463, -20.2726) (-57.7453, -19.0761) (-57.3075, -17.9961) (-56.8206, -17.0415) (-56.2779, -16.2176) (-55.7966, -15.6643) (-55.4088, -15.309) (-55.1382, -15.0986) (-55, -15) knots -1 -1 -1 -1 -1 -1 -0.966667 -0.933333 -0.9 -0.866667 -0.833333 -0.8 -0.766667 -0.733333 -0.7 -0.666667 -0.633333 -0.6 -0.566667 -0.533333 -0.5 -0.466667 -0.433333 -0.4 -0.366667 -0.333333 -0.3 -0.266667 -0.233333 -0.2 -0.166667 -0.133333 -0.1 -0.066667 -0.033333 0 0 0 0 0 0
  spline S14 degree 5 poles (-55, -15) (-54.8618, -15.0986) (-54.5912, -15.309) (-54.2034, -15.6643) (-53.7221, -16.2176) (-53.1794, -17.0415) (-52.6925, -17.9961) (-52.2547, -19.0761) (-51.8537, -20.2726) (-51.4726, -21.5702) (-51.0928, -22.9453) (-50.6957, -24.3634) (-50.2655, -25.777) (-49.7912, -27.1236) (-49.2698, -28.3211) (-48.7063, -29.2738) (-48.1114, -29.8918) (-47.5, -30.1073) (-46.8886, -29.8918) (-46.2937, -29.2738) (-45.7302, -28.3211) (-45.2088, -27.1236) (-44.7345, -25.777) (-44.3043, -24.3634) (-43.9072, -22.9453) (-43.5274, -21.5702) (-43.1463, -20.2726) (-42.7453, -19.0761) (-42.3075, -17.9961) (-41.8206, -17.0415) (-41.2779, -16.2176) (-40.7966, -15.6643) (-40.4088, -15.309) (-40.1382, -15.0986) (-40, -15) knots -1 -1 -1 -1 -1 -1 -0.966667 -0.933333 -0.9 -0.866667 -0.833333 -0.8 -0.766667 -0.733333 -0.7 -0.666667 -0.633333 -0.6 -0.566667 -0.533333 -0.5 -0.466667 -0.433333 -0.4 -0.366667 -0.333333 -0.3 -0.266667 -0.233333 -0.2 -0.166667 -0.133333 -0.1 -0.066667 -0.033333 0 0 0 0 0 0
  spline S15 degree 5 poles (-40, -15) (-39.8618, -15.0986) (-39.5912, -15.309) (-39.2034, -15.6643) (-38.7221, -16.2176) (-38.1794, -17.0415) (-37.6925, -17.9961) (-37.2547, -19.0761) (-36.8537, -20.2726) (-36.4726, -21.5702) (-36.0928, -22.9453) (-35.6957, -24.3634) (-35.2655, -25.777) (-34.7912, -27.1236) (-34.2698, -28.3211) (-33.7063, -29.2738) (-33.1114, -29.8918) (-32.5, -30.1073) (-31.8886, -29.8918) (-31.2937, -29.2738) (-30.7302, -28.3211) (-30.2088, -27.1236) (-29.7345, -25.777) (-29.3043, -24.3634) (-28.9072, -22.9453) (-28.5274, -21.5702) (-28.1463, -20.2726) (-27.7453, -19.0761) (-27.3075, -17.9961) (-26.8206, -17.0415) (-26.2779, -16.2176) (-25.7966, -15.6643) (-25.4088, -15.309) (-25.1382, -15.0986) (-25, -15) knots -1 -1 -1 -1 -1 -1 -0.966667 -0.933333 -0.9 -0.866667 -0.833333 -0.8 -0.766667 -0.733333 -0.7 -0.666667 -0.633333 -0.6 -0.566667 -0.533333 -0.5 -0.466667 -0.433333 -0.4 -0.366667 -0.333333 -0.3 -0.266667 -0.233333 -0.2 -0.166667 -0.133333 -0.1 -0.066667 -0.033333 0 0 0 0 0 0
  spline S16 degree 5 poles (-25, -15) (-24.8618, -15.0986) (-24.5912, -15.309) (-24.2034, -15.6643) (-23.7221, -16.2176) (-23.1794, -17.0415) (-22.6925, -17.9961) (-22.2547, -19.0761) (-21.8537, -20.2726) (-21.4726, -21.5702) (-21.0928, -22.9453) (-20.6957, -24.3634) (-20.2655, -25.777) (-19.7912, -27.1236) (-19.2698, -28.3211) (-18.7063, -29.2738) (-18.1114, -29.8918) (-17.5, -30.1073) (-16.8886, -29.8918) (-16.2937, -29.2738) (-15.7302, -28.3211) (-15.2088, -27.1236) (-14.7345, -25.777) (-14.3043, -24.3634) (-13.9072, -22.9453) (-13.5274, -21.5702) (-13.1463, -20.2726) (-12.7453, -19.0761) (-12.3075, -17.9961) (-11.8206, -17.0415) (-11.2779, -16.2176) (-10.7966, -15.6643) (-10.4088, -15.309) (-10.1382, -15.0986) (-10, -15) knots -1 -1 -1 -1 -1 -1 -0.966667 -0.933333 -0.9 -0.866667 -0.833333 -0.8 -0.766667 -0.733333 -0.7 -0.666667 -0.633333 -0.6 -0.566667 -0.533333 -0.5 -0.466667 -0.433333 -0.4 -0.366667 -0.333333 -0.3 -0.266667 -0.233333 -0.2 -0.166667 -0.133333 -0.1 -0.066667 -0.033333 0 0 0 0 0 0
  line L31 (-267, -13) -> (-264.3599, -13)
  spline S17 degree 3 poles (-250, -12.5435) (-249.6129, -12.8196) (-249.2258, -13.0956) (-248.8387, -13.3717) (-247.4048, -14.3943) (-246.3881, -15.9477) (-245.6468, -17.7479) (-244.9554, -19.4267) (-244.4675, -21.3627) (-243.9195, -23.2775) (-243.5808, -24.4611) (-243.2149, -25.6362) (-242.8326, -26.5675) (-242.7208, -26.8397) (-242.6088, -27.0889) (-242.5, -27.3069) knots -1.056001 -1.056001 -1.056001 -1.056001 -1 -1 -1 -0.851292 -0.851292 -0.851292 -0.71262 -0.71262 -0.71262 -0.626906 -0.626906 -0.626906 -0.601856 -0.601856 -0.601856 -0.601856
  spline S18 degree 3 poles (-242.5, -27.3069) (-242.0881, -26.4817) (-241.6514, -25.2172) (-241.2668, -23.9183) (-240.7129, -22.0478) (-240.237, -20.0931) (-239.6002, -18.3797) (-238.9085, -16.5186) (-237.986, -14.8851) (-236.6355, -13.7409) (-236.4823, -13.6111) (-236.3242, -13.4878) (-236.1613, -13.3717) (-235.7742, -13.0956) (-235.3871, -12.8196) (-235, -12.5435) knots -0.398144 -0.398144 -0.398144 -0.398144 -0.30293 -0.30293 -0.30293 -0.165823 -0.165823 -0.165823 -0.016893 -0.016893 -0.016893 0 0 0 0.056001 0.056001 0.056001 0.056001
  spline S19 degree 3 poles (-235, -12.5435) (-234.6129, -12.8196) (-234.2258, -13.0956) (-233.8387, -13.3717) (-232.4048, -14.3943) (-231.3881, -15.9477) (-230.6468, -17.7479) (-229.9554, -19.4267) (-229.4675, -21.3627) (-228.9195, -23.2775) (-228.5808, -24.4611) (-228.2149, -25.6362) (-227.8326, -26.5675) (-227.7208, -26.8397) (-227.6088, -27.0889) (-227.5, -27.3069) knots -1.056001 -1.056001 -1.056001 -1.056001 -1 -1 -1 -0.851292 -0.851292 -0.851292 -0.71262 -0.71262 -0.71262 -0.626906 -0.626906 -0.626906 -0.601856 -0.601856 -0.601856 -0.601856
  spline S20 degree 3 poles (-227.5, -27.3069) (-227.0881, -26.4817) (-226.6514, -25.2172) (-226.2668, -23.9183) (-225.7129, -22.0478) (-225.237, -20.0931) (-224.6002, -18.3797) (-223.9085, -16.5186) (-222.986, -14.8851) (-221.6355, -13.7409) (-221.4823, -13.6111) (-221.3242, -13.4878) (-221.1613, -13.3717) (-220.7742, -13.0956) (-220.3871, -12.8196) (-220, -12.5435) knots -0.398144 -0.398144 -0.398144 -0.398144 -0.30293 -0.30293 -0.30293 -0.165823 -0.165823 -0.165823 -0.016893 -0.016893 -0.016893 0 0 0 0.056001 0.056001 0.056001 0.056001
  spline S21 degree 3 poles (-220, -12.5435) (-219.6129, -12.8196) (-219.2258, -13.0956) (-218.8387, -13.3717) (-217.4048, -14.3943) (-216.3881, -15.9477) (-215.6468, -17.7479) (-214.9554, -19.4267) (-214.4675, -21.3627) (-213.9195, -23.2775) (-213.5808, -24.4611) (-213.2149, -25.6362) (-212.8326, -26.5675) (-212.7208, -26.8397) (-212.6088, -27.0889) (-212.5, -27.3069) knots -1.056001 -1.056001 -1.056001 -1.056001 -1 -1 -1 -0.851292 -0.851292 -0.851292 -0.71262 -0.71262 -0.71262 -0.626906 -0.626906 -0.626906 -0.601856 -0.601856 -0.601856 -0.601856
  spline S22 degree 3 poles (-212.5, -27.3069) (-212.0881, -26.4817) (-211.6514, -25.2172) (-211.2668, -23.9183) (-210.7129, -22.0478) (-210.237, -20.0931) (-209.6002, -18.3797) (-208.9085, -16.5186) (-207.986, -14.8851) (-206.6355, -13.7409) (-206.4823, -13.6111) (-206.3242, -13.4878) (-206.1613, -13.3717) (-205.7742, -13.0956) (-205.3871, -12.8196) (-205, -12.5435) knots -0.398144 -0.398144 -0.398144 -0.398144 -0.30293 -0.30293 -0.30293 -0.165823 -0.165823 -0.165823 -0.016893 -0.016893 -0.016893 0 0 0 0.056001 0.056001 0.056001 0.056001
  spline S23 degree 3 poles (-205, -12.5435) (-204.6129, -12.8196) (-204.2258, -13.0956) (-203.8387, -13.3717) (-202.4048, -14.3943) (-201.3881, -15.9477) (-200.6468, -17.7479) (-199.9554, -19.4267) (-199.4675, -21.3627) (-198.9195, -23.2775) (-198.5808, -24.4611) (-198.2149, -25.6362) (-197.8326, -26.5675) (-197.7208, -26.8397) (-197.6088, -27.0889) (-197.5, -27.3069) knots -1.056001 -1.056001 -1.056001 -1.056001 -1 -1 -1 -0.851292 -0.851292 -0.851292 -0.71262 -0.71262 -0.71262 -0.626906 -0.626906 -0.626906 -0.601856 -0.601856 -0.601856 -0.601856
  spline S24 degree 3 poles (-197.5, -27.3069) (-197.0881, -26.4817) (-196.6514, -25.2172) (-196.2668, -23.9183) (-195.7129, -22.0478) (-195.237, -20.0931) (-194.6002, -18.3797) (-193.9085, -16.5186) (-192.986, -14.8851) (-191.6355, -13.7409) (-191.4823, -13.6111) (-191.3242, -13.4878) (-191.1613, -13.3717) (-190.7742, -13.0956) (-190.3871, -12.8196) (-190, -12.5435) knots -0.398144 -0.398144 -0.398144 -0.398144 -0.30293 -0.30293 -0.30293 -0.165823 -0.165823 -0.165823 -0.016893 -0.016893 -0.016893 0 0 0 0.056001 0.056001 0.056001 0.056001
  spline S25 degree 3 poles (-190, -12.5435) (-189.6129, -12.8196) (-189.2258, -13.0956) (-188.8387, -13.3717) (-187.4048, -14.3943) (-186.3881, -15.9477) (-185.6468, -17.7479) (-184.9554, -19.4267) (-184.4675, -21.3627) (-183.9195, -23.2775) (-183.5808, -24.4611) (-183.2149, -25.6362) (-182.8326, -26.5675) (-182.7208, -26.8397) (-182.6088, -27.0889) (-182.5, -27.3069) knots -1.056001 -1.056001 -1.056001 -1.056001 -1 -1 -1 -0.851292 -0.851292 -0.851292 -0.71262 -0.71262 -0.71262 -0.626906 -0.626906 -0.626906 -0.601856 -0.601856 -0.601856 -0.601856
  spline S26 degree 3 poles (-182.5, -27.3069) (-182.0881, -26.4817) (-181.6514, -25.2172) (-181.2668, -23.9183) (-180.7129, -22.0478) (-180.237, -20.0931) (-179.6002, -18.3797) (-178.9085, -16.5186) (-177.986, -14.8851) (-176.6355, -13.7409) (-176.4823, -13.6111) (-176.3242, -13.4878) (-176.1613, -13.3717) (-175.7742, -13.0956) (-175.3871, -12.8196) (-175, -12.5435) knots -0.398144 -0.398144 -0.398144 -0.398144 -0.30293 -0.30293 -0.30293 -0.165823 -0.165823 -0.165823 -0.016893 -0.016893 -0.016893 0 0 0 0.056001 0.056001 0.056001 0.056001
  spline S27 degree 3 poles (-175, -12.5435) (-174.6129, -12.8196) (-174.2258, -13.0956) (-173.8387, -13.3717) (-172.4048, -14.3943) (-171.3881, -15.9477) (-170.6468, -17.7479) (-169.9554, -19.4267) (-169.4675, -21.3627) (-168.9195, -23.2775) (-168.5808, -24.4611) (-168.2149, -25.6362) (-167.8326, -26.5675) (-167.7208, -26.8397) (-167.6088, -27.0889) (-167.5, -27.3069) knots -1.056001 -1.056001 -1.056001 -1.056001 -1 -1 -1 -0.851292 -0.851292 -0.851292 -0.71262 -0.71262 -0.71262 -0.626906 -0.626906 -0.626906 -0.601856 -0.601856 -0.601856 -0.601856
  spline S28 degree 3 poles (-167.5, -27.3069) (-167.0881, -26.4817) (-166.6514, -25.2172) (-166.2668, -23.9183) (-165.7129, -22.0478) (-165.237, -20.0931) (-164.6002, -18.3797) (-163.9085, -16.5186) (-162.986, -14.8851) (-161.6355, -13.7409) (-161.4823, -13.6111) (-161.3242, -13.4878) (-161.1613, -13.3717) (-160.7742, -13.0956) (-160.3871, -12.8196) (-160, -12.5435) knots -0.398144 -0.398144 -0.398144 -0.398144 -0.30293 -0.30293 -0.30293 -0.165823 -0.165823 -0.165823 -0.016893 -0.016893 -0.016893 0 0 0 0.056001 0.056001 0.056001 0.056001
  spline S29 degree 3 poles (-160, -12.5435) (-159.6129, -12.8196) (-159.2258, -13.0956) (-158.8387, -13.3717) (-157.4048, -14.3943) (-156.3881, -15.9477) (-155.6468, -17.7479) (-154.9554, -19.4267) (-154.4675, -21.3627) (-153.9195, -23.2775) (-153.5808, -24.4611) (-153.2149, -25.6362) (-152.8326, -26.5675) (-152.7208, -26.8397) (-152.6088, -27.0889) (-152.5, -27.3069) knots -1.056001 -1.056001 -1.056001 -1.056001 -1 -1 -1 -0.851292 -0.851292 -0.851292 -0.71262 -0.71262 -0.71262 -0.626906 -0.626906 -0.626906 -0.601856 -0.601856 -0.601856 -0.601856